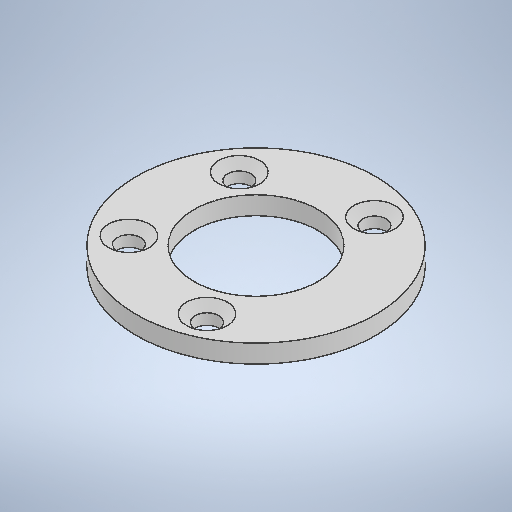
# Autodesk Inventor part: Simple_Mouting_Bracket
Saved by Autodesk Inventor 2026.2 (Build 302298000, 298)
## iProperties
Created: 2026-03-06
Part Number: Simple_Mouting_Bracket
Material: Generic
Document SubType Name: Modeling
Designer: Paco Ariel
Density: 1 g/cm^3
Appearance: Default
Author: Paco Ariel
Autodesk Inventor part; units mm, degrees
ref_plane "YZ Plane" through (0, 0, 0) normal (1, 0, 0) x (0, 1, 0)
ref_plane "XZ Plane" through (0, 0, 0) normal (0, 1, 0) x (-1, 0, 0)
ref_plane "XY Plane" through (0, 0, 0) normal (0, 0, 1) x (1, 0, 0)
sketch "Sketch1" plane through (0, 0, 0) normal (0, 1, 0) x (-1, 0, 0)
  circle A0 centre (0, 0) radius 16.45
  circle A1 centre (0, 0) radius 8.55
  dimension "d0" = 32.9
  dimension "d1" = 17.1
  constraints: 2 centre point, 2 coincident
  measures "d0" diameter of A0
  measures "d1" diameter of A1
extrude "Extrusion1" add sketch "Sketch1" along normal blind 2.5
sketch "Sketch2" plane through (0, 2.5, 0) normal (0, 1, 0) x (1, 0, 0)
  circle A0 centre (0, 0) radius 12.475
  line L0 (0, 0) -> (4.774, -11.5254)
  line L1 (0, 0) -> (21.8352, 0) construction
  line L2 (0, 0) -> (4.774, 11.5254)
  line L3 (0, 0) -> (76.5, 0) construction
  point P0 (-9.8971, -7.5943)
  point P1 (-9.8971, 7.5943)
  point P2 (4.774, 11.5254)
  dimension "d4" = 24.95
  dimension "d5" = 67.5
  dimension "d7" = 67.5
  dimension "d10" = 225
  constraints: 8 end point, 2 coincident, 2 horizontal, 2 point on circle, 1 centre point, 4 other
  measures "d4" diameter of A0
  measures "d5" angle of L0 L1
  measures "d7" angle of L3 L2
hole "Hole1" at (4.774, 2.5, 11.5254) at (-9.8971, 2.5, 7.5943) at (-9.8971, 2.5, -7.5943) at (4.774, 2.5, -11.5254) direction (0, -1, 0) diameter 3.2 depth 4 tip angle 118
chamfer "Chamfer1" distance 1.2 distance2 1 4 edges at (4.774, 2.5, -13.1254) (-9.8971, 2.5, -9.1943) (4.774, 2.5, 9.9254) (-9.8971, 2.5, 5.9943) measured on face at (-5.8151, 2.5, -10.6262)
body "Solid1"
